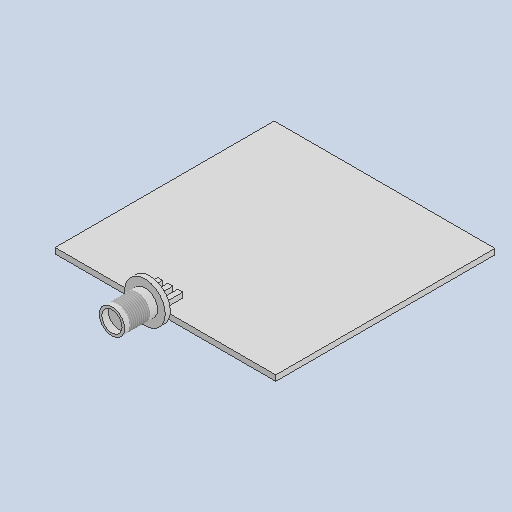
# Autodesk Inventor part: ZED-F9P-02B
Saved by Autodesk Inventor 2025.2 (Build 292293000, 293)
## iProperties
Created: 2025-05-12
Part Number: ZED-F9P-02B
Material: 일반
Document SubType Name: Modeling
Designer: jbhma
Density: 1 g/cm^3
Appearance: 기본값
Author: jbhma
Autodesk Inventor part; units mm, degrees
ref_plane "YZ Plane" through (0, 0, 0) normal (1, 0, 0) x (0, 1, 0)
ref_plane "XZ Plane" through (0, 0, 0) normal (0, 1, 0) x (-1, 0, 0)
ref_plane "XY Plane" through (0, 0, 0) normal (0, 0, 1) x (1, 0, 0)
sketch "스케치1" plane through (0, 0, 0) normal (0, 1, 0) x (-1, 0, 0)
  line L0 (-217.5, -432) -> (217.5, -432)
  line L1 (217.5, -432) -> (217.5, 0)
  line L2 (217.5, 0) -> (-217.5, 0)
  line L3 (-217.5, 0) -> (-217.5, -432)
  point P0 (0, 0)
  point P1 (0, 0)
  dimension "d0" = 435
  dimension "d1" = 432
  constraints: 8 end point, 2 parallel, 1 coincident, 1 horizontal, 1 midpoint, 1 perpendicular
  measures "d0" distance of L2.end L1.end
  measures "d1" distance of L1.end L0.end
extrude "돌출1" add sketch "스케치1" along normal blind 11
sketch "스케치2" plane through (0, 11, 0) normal (0, 1, 0) x (1, 0, 0)
  line L0 (-217.5, 432) -> (-217.5, 0) projected
  line L1 (-217.5, 0) -> (217.5, 0) projected
  line L2 (217.5, 0) -> (217.5, 432) projected
  line L3 (217.5, 432) -> (-217.5, 432) projected
  line L4 (-55.5, 0) -> (-45.5, 0)
  line L5 (-45.5, 0) -> (-45.5, 40)
  line L6 (-45.5, 40) -> (-55.5, 40)
  line L7 (-55.5, 40) -> (-55.5, 0)
  line L8 (-35.5, 0) -> (-25.5, 0)
  line L9 (-25.5, 0) -> (-25.5, 40)
  line L10 (-25.5, 40) -> (-35.5, 40)
  line L11 (-35.5, 40) -> (-35.5, 0)
  line L12 (-15.5, 0) -> (-5.5, 0)
  line L13 (-5.5, 0) -> (-5.5, 40)
  line L14 (-5.5, 40) -> (-15.5, 40)
  line L15 (-15.5, 40) -> (-15.5, 0)
  point P0 (0, 0)
  dimension "d5" = 10
  dimension "d6" = 40
  dimension "d7" = 10
  dimension "d8" = 10
  dimension "d9" = 40
  dimension "d10" = 10
  dimension "d11" = 10
  dimension "d12" = 40
  dimension "d13" = 223
  constraints: 24 end point, 6 parallel, 3 horizontal, 3 perpendicular, 3 point on line
  measures "d5" distance of L6.end L5.end
  measures "d6" distance of L5.end L4.end
  measures "d7" distance of L4.end L8.start
  measures "d8" distance of L10.end L9.end
  measures "d9" distance of L9.end L8.end
  measures "d10" distance of L8.end L12.start
  measures "d11" distance of L14.end L13.end
  measures "d12" distance of L13.end L12.end
  measures "d13" distance between parallel lines of L2 L13
extrude "돌출2" add sketch "스케치2" along normal blind 10 contours L7 L6 L5 L1 | L1 L15 L14 L13 | L11 L10 L9 L1
sketch "스케치3" plane through (-217.5, 0, 0) normal (0, 0, 1) x (1, 0, 0)
  line L0 (0, 0) -> (435, 0) projected
  line L1 (435, 0) -> (435, 11) projected
  line L2 (212, 11) -> (435, 11) projected
  line L3 (212, 11) -> (212, 21) projected
  line L4 (202, 21) -> (212, 21) projected
  line L5 (202, 11) -> (202, 21) projected
  line L6 (192, 11) -> (202, 11) projected
  line L7 (192, 11) -> (192, 21) projected
  line L8 (182, 21) -> (192, 21) projected
  line L9 (182, 11) -> (182, 21) projected
  line L10 (172, 11) -> (182, 11) projected
  line L11 (172, 11) -> (172, 21) projected
  line L12 (162, 21) -> (172, 21) projected
  line L13 (162, 11) -> (162, 21) projected
  line L14 (0, 11) -> (162, 11) projected
  line L15 (0, 0) -> (0, 11) projected
  circle A0 centre (187, 16) radius 40
  point P0 (217.5, 0)
  dimension "d16" = 80
  constraints: 1 centre point
  measures "d16" diameter of A0
extrude "돌출3" add sketch "스케치3" along normal blind 10 contours A0 L14 L13 L12 L11 L10 L9 L8 L7 L6 L5 L4 L3 L2 L0 | L0 A0 | A0 L2 L3 L4 L5 L6 L7 L8 L9 L10 L11 L12 L13 L14
sketch "스케치4" plane through (-30.5, 16, 10) normal (0, 0, 1) x (1, 0, 0)
  circle A0 centre (0, 0) radius 40 projected
  circle A1 centre (0, 0) radius 25
  point P0 (30.5, -16)
  dimension "d19" = 50
  constraints: 1 centre point, 1 coincident
  measures "d19" diameter of A1
extrude "돌출4" add sketch "스케치4" along normal blind 65 contours A1
thread "스레드1" size "M50x4" class "6g" standard "ISO Metric profile" length 40 offset 15
sketch "스케치5" plane through (-30.5, 16, 75) normal (0, 0, 1) x (1, 0, 0)
  circle A0 centre (0, 0) radius 25 projected
  circle A1 centre (0, 0) radius 20
  point P0 (30.5, -16)
  dimension "d24" = 40
  constraints: 1 centre point, 1 coincident
  measures "d24" diameter of A1
extrude "돌출5" cut sketch "스케치5" against normal blind 13 contours A1
